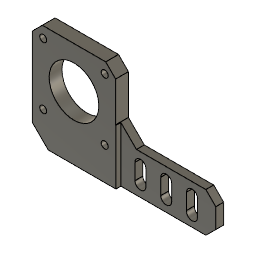
Main Assembly (Autodesk Fusion 360 archive; units mm, degrees)
design "Motor Mount"
Autodesk Fusion 360 part; units mm, degrees
sketch "Sketch1" plane through (0, 0, 0) normal (0, 1, 0) x (1, 0, 0)
  line L0 (0, 0) -> (42, 0) construction
  line L1 (42, 0) -> (42, -42) construction
  line L2 (42, -42) -> (0, -42)
  line L3 (0, -42) -> (0, 0)
  line L4 (5.5, -5.5) -> (36.5, -5.5) construction
  line L5 (36.5, -5.5) -> (36.5, -36.5) construction
  line L6 (36.5, -36.5) -> (5.5, -36.5) construction
  line L7 (5.5, -36.5) -> (5.5, -5.5) construction
  circle A0 centre (36.5, -36.5) radius 1.75
  circle A1 centre (5.5, -36.5) radius 1.75
  circle A2 centre (5.5, -5.5) radius 1.75
  circle A3 centre (36.5, -5.5) radius 1.75
  line L8 (0, -21) -> (42, -21) construction
  circle A4 centre (21, -21) radius 12.5
  line L9 (0, 0) -> (0, 11)
  line L10 (0, 11) -> (90, 11)
  line L11 (90, 11) -> (90, -9)
  line L12 (90, -9) -> (42, -9)
  line L13 (42, -9) -> (42, -42)
  line L14 (90, 1) -> (42, 1) construction
  line L15 (67.75, -3) -> (62.25, -3) construction
  line L16 (62.25, -3) -> (62.25, 5)
  line L17 (62.25, 5) -> (67.75, 5) construction
  line L18 (67.75, 5) -> (67.75, -3)
  line L19 (67.75, -3) -> (62.25, 5) construction
  line L20 (62.25, -3) -> (67.75, 5) construction
  line L21 (65, 1) -> (52, 1)
  line L22 (65, 1) -> (78, 1)
  line L23 (54.75, -3) -> (49.25, -3) construction
  line L24 (49.25, -3) -> (49.25, 5)
  line L25 (49.25, 5) -> (54.75, 5) construction
  line L26 (54.75, 5) -> (54.75, -3)
  line L27 (54.75, -3) -> (49.25, 5) construction
  line L28 (49.25, -3) -> (54.75, 5) construction
  line L29 (75.25, -3) -> (80.75, -3) construction
  line L30 (80.75, -3) -> (80.75, 5)
  line L31 (80.75, 5) -> (75.25, 5) construction
  line L32 (75.25, 5) -> (75.25, -3)
  line L33 (75.25, -3) -> (80.75, 5) construction
  line L34 (80.75, -3) -> (75.25, 5) construction
  arc A5 (54.75, 5) -> (49.25, 5) centre (52, 5) ccw
  arc A6 (49.25, -3) -> (54.75, -3) centre (52, -3) ccw
  arc A7 (67.75, 5) -> (62.25, 5) centre (65, 5) ccw
  arc A8 (62.25, -3) -> (67.75, -3) centre (65, -3) ccw
  arc A9 (75.25, -3) -> (80.75, -3) centre (78, -3) ccw
  arc A10 (80.75, 5) -> (75.25, 5) centre (78, 5.3653) ccw
  point P0 (65, 1)
  point P1 (52, 1)
  point P2 (78, 1)
  dimension "d1" = 42
  dimension "d2" = 42
  dimension "d3" = 5.5
  dimension "d4" = 3.5
  dimension "d5" = 3.5
  dimension "d6" = 3.5
  dimension "d7" = 3.5
  dimension "d12" = 11
  dimension "d13" = 90
  dimension "d14" = 20
  dimension "d15" = 5.5
  dimension "d16" = 13
  dimension "d17" = 13
  dimension "d18" = 5.5
  dimension "d19" = 8
  dimension "d20" = 5.5
  dimension "d21" = 8
  dimension "d24" = 25
  constraint horizontal L0
  constraint vertical L1
  constraint horizontal L2
  constraint vertical L3
  constraint coincident L0.start L3.end
  constraint coincident L5.end L6.start
  constraint coincident L6.end L7.start
  constraint coincident L4.start L7.end
  constraint coincident L4.end L5.start
  constraint midpoint L3 L8.start
  constraint midpoint L1 L8.end
  constraint midpoint L8 A4.centre
  constraint perpendicular L0 L9
  constraint perpendicular L9 L10
  constraint perpendicular L10 L11
  constraint coincident L1 L12.end
  constraint perpendicular L1 L12
  constraint midpoint L11 L14.start
  constraint perpendicular L11 L14
  constraint horizontal L15
  constraint perpendicular L15 L16
  constraint parallel L15 L17
  constraint parallel L16 L18
  constraint coincident L19 P0
  constraint coincident L20 P0
  constraint coincident L14 P0
  constraint coincident P0 L21.start
  constraint perpendicular L16 L21
  constraint perpendicular L18 L22
  constraint horizontal L23
  constraint perpendicular L23 L24
  constraint parallel L23 L25
  constraint parallel L24 L26
  constraint coincident L27 P1
  constraint coincident L28 P1
  constraint coincident P1 L21.end
  constraint horizontal L29
  constraint perpendicular L29 L30
  constraint parallel L29 L31
  constraint parallel L30 L32
  constraint coincident L33 P2
  constraint coincident L34 P2
  constraint coincident P2 L22.end
  constraint tangent L26 A5
  constraint tangent L26 A6
  constraint tangent L18 A7
  constraint tangent L18 A8
  constraint tangent L30 A9
  measures "d1" distance of L0.start L0.end
  measures "d2" distance of L0.start L2.end
  measures "d4" diameter of A0
  measures "d5" diameter of A1
  measures "d6" diameter of A2
  measures "d7" diameter of A3
  measures "d12" distance of L0.start L9.end
  measures "d13" distance of L9.end L10.end
  measures "d14" distance of L10.end L11.end
  measures "d15" distance of L16.end L17.end
  measures "d16" distance of P0 P1
  measures "d17" distance of P0 P2
  measures "d18" distance of L24.end L25.end
  measures "d19" distance of L23.end L24.end
  measures "d20" distance of L30.end L31.end
  measures "d21" distance of L29.end L30.end
  measures "d24" diameter of A4
extrude "Extrude1" add sketch "Sketch1" along normal blind 6.5
chamfer "Chamfer1" distance 8 angle 45 2 edges at (42, 3.25, 9) (0, 3.25, -11)
chamfer "Chamfer2" distance 5 angle 45 4 edges at (90, 3.25, 9) (90, 3.25, -11) (42, 3.25, 42) (0, 3.25, 42)
sketch "Sketch2" plane through (0, 0, -11) normal (0, 0, -1) x (1, 0, 0)
  line L0 (85, -6.5) -> (85, 0)
  line L1 (85, 0) -> (8, 0)
  line L2 (8, 0) -> (8, -6.5)
  line L3 (8, -6.5) -> (85, -6.5)
  line L4 (90, 0) -> (42.1425, 0)
  line L5 (42.1425, 0) -> (42.1425, -2.5)
  line L6 (42.1425, -2.5) -> (90, -2.5)
  line L7 (90, -2.5) -> (90, 0)
  dimension "d25" = 2.5
  constraint horizontal L4
  constraint vertical L5
  constraint horizontal L6
  constraint vertical L7
  measures "d25" distance of L4.start L6.end
extrude "Extrude3" cut sketch "Sketch2" against normal blind 36 contours L0 L1 L4 L5 L6 | L0 L4 L6 L7
equation "d25 = 6.5 mm - 4 mm"

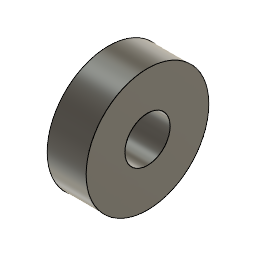
design "Bearing"
Autodesk Fusion 360 part; units mm, degrees
sketch "Sketch1" plane through (0, 0, 0) normal (1, 0, 0) x (0, 1, 0)
  circle A0 centre (0, 0) radius 11
  dimension "d1" = 22
  constraint coincident A0.centre origin
  measures "d1" diameter of A0
extrude "Extrude1" add sketch "Sketch1" along normal blind 7
sketch "Sketch2" plane through (7, 0, 0) normal (1, 0, 0) x (0, 1, 0)
  circle A0 centre (0, 0) radius 11
  circle A1 centre (0, 0) radius 4.05
  dimension "d4" = 8.1
  constraint concentric A0 A1
  measures "d4" diameter of A1
extrude "Extrude2" cut sketch "Sketch2" against normal blind 30 contours A1

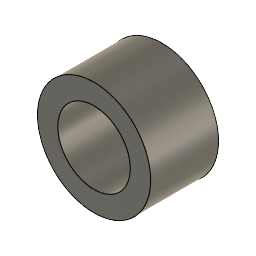
design "Bushings"
Autodesk Fusion 360 part; units mm, degrees
sketch "Sketch1" plane through (0, 0, 0) normal (0, 1, 0) x (1, 0, 0)
  circle A0 centre (0, 0) radius 4
  circle A1 centre (0, 0) radius 6.25
  dimension "d1" = 8
  dimension "d2" = 12.5
  constraint coincident A0.centre A1.centre
  measures "d1" diameter of A0
  measures "d2" diameter of A1
extrude "Extrude1" add sketch "Sketch1" along normal blind 7.5
equation "d3 = 5.75 mm + 1.75 mm"

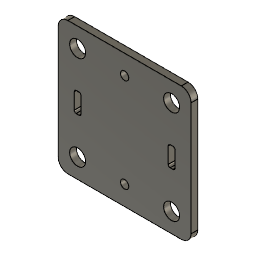
design "Gantry Plate"
Autodesk Fusion 360 part; units mm, degrees
sketch "Sketch1" plane through (0, 0, 0) normal (0, 1, 0) x (1, 0, 0)
  line L0 (0, 0) -> (48.25, 0) construction
  line L1 (48.25, 0) -> (48.25, -48.25) construction
  line L2 (48.25, -48.25) -> (0, -48.25) construction
  line L3 (0, -48.25) -> (0, 0) construction
  line L4 (-5, 10) -> (53.25, 10)
  line L5 (58.25, 5) -> (58.25, -53.25)
  line L6 (53.25, -58.25) -> (-5, -58.25)
  line L7 (-10, -53.25) -> (-10, 5)
  circle A0 centre (48.25, -48.25) radius 4.1
  circle A1 centre (48.25, 0) radius 4.1
  circle A2 centre (0, 0) radius 4.1
  circle A3 centre (0, -48.25) radius 4.1
  line L8 (49, -19) -> (47.5, -19)
  line L9 (46.5, -20) -> (46.5, -28.25)
  line L10 (47.5, -29.25) -> (49, -29.25)
  line L11 (50, -28.25) -> (50, -20)
  line L12 (50, -19) -> (46.5, -29.25) construction
  line L13 (46.5, -19) -> (50, -29.25) construction
  line L14 (0.75, -19) -> (-0.75, -19)
  line L15 (-1.75, -20) -> (-1.75, -28.25)
  line L16 (-0.75, -29.25) -> (0.75, -29.25)
  line L17 (1.75, -28.25) -> (1.75, -20)
  line L18 (1.75, -19) -> (-1.75, -29.25) construction
  line L19 (-1.75, -19) -> (1.75, -29.25) construction
  arc A4 (-10, -53.25) -> (-5, -58.25) centre (-5, -53.25) ccw
  arc A5 (53.25, -58.25) -> (58.25, -53.25) centre (53.25, -53.25) ccw
  arc A6 (58.25, 5) -> (53.25, 10) centre (53.25, 5) ccw
  arc A7 (-5, 10) -> (-10, 5) centre (-5, 5) ccw
  arc A8 (-1.75, -28.25) -> (-0.75, -29.25) centre (-0.75, -28.25) ccw
  arc A9 (0.75, -29.25) -> (1.75, -28.25) centre (0.75, -28.25) ccw
  arc A10 (1.75, -20) -> (0.75, -19) centre (0.75, -20) ccw
  arc A11 (-0.75, -19) -> (-1.75, -20) centre (-0.75, -20) ccw
  arc A12 (46.5, -28.25) -> (47.5, -29.25) centre (47.5, -28.25) ccw
  arc A13 (49, -29.25) -> (50, -28.25) centre (49, -28.25) ccw
  arc A14 (50, -20) -> (49, -19) centre (49, -20) ccw
  arc A15 (47.5, -19) -> (46.5, -20) centre (47.5, -20) ccw
  point P0 (48.25, -24.125)
  point P1 (0, -24.125)
  dimension "d1" = 48.25
  dimension "d2" = 48.25
  dimension "d4" = 8.2
  dimension "d5" = 8.2
  dimension "d6" = 8.2
  dimension "d7" = 8.2
  dimension "d8" = 3.5
  dimension "d9" = 10.25
  dimension "d10" = 3.5
  dimension "d11" = 10.25
  dimension "d12" = 5
  dimension "d13" = 1
  dimension "d14" = 1
  constraint horizontal L0
  constraint vertical L1
  constraint horizontal L2
  constraint vertical L3
  constraint coincident L0.start L3.end
  constraint coincident L1.end L2.start
  constraint coincident L0.end L1.start
  constraint coincident L2.end L3.start
  constraint horizontal L8
  constraint perpendicular L8 L9
  constraint parallel L8 L10
  constraint parallel L9 L11
  constraint coincident L12 P0
  constraint coincident L13 P0
  constraint midpoint L1 P0
  constraint horizontal L14
  constraint perpendicular L14 L15
  constraint parallel L14 L16
  constraint parallel L15 L17
  constraint coincident L18 P1
  constraint coincident L19 P1
  constraint midpoint L3 P1
  constraint tangent L6 A4
  constraint tangent L7 A4
  constraint tangent L6 A5
  constraint tangent L5 A5
  constraint equal A4 A5
  constraint tangent L5 A6
  constraint tangent L4 A6
  constraint equal A4 A6
  constraint tangent L4 A7
  constraint tangent L7 A7
  constraint equal A4 A7
  constraint coincident L18.end L16
  constraint coincident L18.end L15
  constraint tangent L16 A8
  constraint tangent L15 A8
  constraint coincident L19.end L17
  constraint coincident L19.end L16
  constraint tangent L17 A9
  constraint tangent L16 A9
  constraint equal A8 A9
  constraint coincident L18.start L17
  constraint coincident L18.start L14
  constraint tangent L17 A10
  constraint tangent L14 A10
  constraint equal A8 A10
  constraint coincident L19.start L14
  constraint coincident L19.start L15
  constraint tangent L14 A11
  constraint tangent L15 A11
  constraint equal A8 A11
  constraint coincident L12.end L10
  constraint coincident L12.end L9
  constraint tangent L10 A12
  constraint tangent L9 A12
  constraint coincident L13.end L11
  constraint coincident L13.end L10
  constraint tangent L11 A13
  constraint tangent L10 A13
  constraint equal A12 A13
  constraint coincident L12.start L11
  constraint coincident L12.start L8
  constraint tangent L11 A14
  constraint tangent L8 A14
  constraint equal A12 A14
  constraint coincident L13.start L8
  constraint coincident L13.start L9
  constraint tangent L8 A15
  constraint tangent L9 A15
  constraint equal A12 A15
  measures "d1" distance of L0.start L0.end
  measures "d2" distance of L0.start L2.end
  measures "d4" diameter of A0
  measures "d5" diameter of A1
  measures "d6" diameter of A2
  measures "d7" diameter of A3
  measures "d8" distance of L12.end L13.end
  measures "d9" distance of L13.start L12.end
  measures "d10" distance of L18.end L19.end
  measures "d11" distance of L19.start L18.end
  measures "d12" radius of A4
  measures "d13" radius of A8
  measures "d14" radius of A12
extrude "Extrude1" add sketch "Sketch1" along normal blind 3.5
sketch "Sketch2" plane through (0, 0, 0) normal (0, -1, 0) x (1, 0, 0)
  circle A0 centre (0, 0) radius 4.1
  arc A1 (46.5, 20) -> (47.5, 19) centre (47.5, 20) ccw
  line L0 (46.5, 20) -> (46.5, 28.25)
  arc A2 (47.5, 29.25) -> (46.5, 28.25) centre (47.5, 28.25) ccw
  line L1 (47.5, 29.25) -> (49, 29.25)
  arc A3 (50, 28.25) -> (49, 29.25) centre (49, 28.25) ccw
  line L2 (50, 28.25) -> (50, 20)
  arc A4 (49, 19) -> (50, 20) centre (49, 20) ccw
  line L3 (49, 19) -> (47.5, 19)
  circle A5 centre (0, 48.25) radius 4.1
  circle A6 centre (48.25, 0) radius 4.1
  arc A7 (-1.75, 20) -> (-0.75, 19) centre (-0.75, 20) ccw
  line L4 (-1.75, 20) -> (-1.75, 28.25)
  arc A8 (-0.75, 29.25) -> (-1.75, 28.25) centre (-0.75, 28.25) ccw
  line L5 (-0.75, 29.25) -> (0.75, 29.25)
  arc A9 (1.75, 28.25) -> (0.75, 29.25) centre (0.75, 28.25) ccw
  line L6 (1.75, 28.25) -> (1.75, 20)
  arc A10 (0.75, 19) -> (1.75, 20) centre (0.75, 20) ccw
  line L7 (0.75, 19) -> (-0.75, 19)
  circle A11 centre (48.25, 48.25) radius 4.1
  arc A12 (53.25, -10) -> (58.25, -5) centre (53.25, -5) ccw
  line L8 (58.25, -5) -> (58.25, 53.25)
  arc A13 (58.25, 53.25) -> (53.25, 58.25) centre (53.25, 53.25) ccw
  line L9 (53.25, 58.25) -> (-5, 58.25)
  arc A14 (-5, 58.25) -> (-10, 53.25) centre (-5, 53.25) ccw
  line L10 (-10, 53.25) -> (-10, -5)
  arc A15 (-10, -5) -> (-5, -10) centre (-5, -5) ccw
  line L11 (-5, -10) -> (53.25, -10)
  line L12 (0, 48.25) -> (48.25, 48.25) construction
  line L13 (48.25, 0) -> (0, 0) construction
  circle A16 centre (24.125, 0) radius 2.125
  circle A17 centre (24.125, 48.25) radius 2.125
  dimension "d17" = 4.25
  dimension "d18" = 4.25
  constraint coincident A5.centre L12.start
  constraint coincident A11.centre L12.end
  constraint coincident A6.centre L13.start
  constraint coincident A0.centre L13.end
  constraint midpoint L13 A16.centre
  constraint midpoint L12 A17.centre
  measures "d17" diameter of A16
  measures "d18" diameter of A17
extrude "Extrude2" cut sketch "Sketch2" against normal blind 21 contours A16 | A17
sketch "Sketch3" plane through (0, 0, 0) normal (0, 1, 0) x (1, 0, 0)

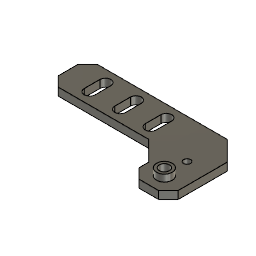
design "Idler Holder Bottom"
Autodesk Fusion 360 part; units mm, degrees
sketch "Sketch1" plane through (0, 0, 0) normal (0, 0, 1) x (1, 0, 0)
  line L0 (0, 0) -> (0, -20)
  line L1 (0, 0) -> (81, 0)
  line L2 (81, 0) -> (81, -40)
  line L3 (81, -40) -> (61, -40)
  line L4 (0, -20) -> (61, -20)
  line L5 (61, -20) -> (61, -40)
  line L6 (71, -40) -> (71, 0)
  circle A0 centre (71, -32) radius 2.6
  line L7 (0, -10) -> (61, -10) construction
  line L8 (27.75, -6) -> (33.25, -6) construction
  line L9 (33.25, -6) -> (33.25, -14)
  line L10 (33.25, -14) -> (27.75, -14) construction
  line L11 (27.75, -14) -> (27.75, -6)
  line L12 (27.75, -6) -> (33.25, -14) construction
  line L13 (33.25, -6) -> (27.75, -14) construction
  line L14 (17.75, -6) -> (12.25, -6) construction
  line L15 (12.25, -6) -> (12.25, -14)
  line L16 (12.25, -14) -> (17.75, -14) construction
  line L17 (17.75, -14) -> (17.75, -6)
  line L18 (17.75, -6) -> (12.25, -14) construction
  line L19 (12.25, -6) -> (17.75, -14) construction
  line L20 (48.75, -6) -> (43.25, -6) construction
  line L21 (43.25, -6) -> (43.25, -14)
  line L22 (43.25, -14) -> (48.75, -14) construction
  line L23 (48.75, -14) -> (48.75, -6)
  line L24 (48.75, -6) -> (43.25, -14) construction
  line L25 (43.25, -6) -> (48.75, -14) construction
  arc A1 (17.75, -6) -> (12.25, -6) centre (15, -6) ccw
  arc A2 (33.25, -6) -> (27.75, -6) centre (30.5, -6) ccw
  arc A3 (48.75, -6) -> (43.25, -6) centre (46, -6) ccw
  arc A4 (43.25, -14) -> (48.75, -14) centre (46, -14) ccw
  arc A5 (27.75, -14) -> (33.25, -14) centre (30.5, -14) ccw
  arc A6 (12.25, -14) -> (17.75, -14) centre (15, -14) ccw
  point P0 (30.5, -10)
  point P1 (15, -10)
  point P2 (46, -10)
  dimension "d1" = 20
  dimension "d2" = 81
  dimension "d3" = 40
  dimension "d4" = 20
  dimension "d5" = 61
  dimension "d11" = 5.2
  dimension "d12" = 32
  dimension "d16" = 5.5
  dimension "d17" = 8
  dimension "d18" = 5.5
  dimension "d19" = 5.5
  dimension "d20" = 8
  dimension "d23" = 34.509
  dimension "d24" = 10
  dimension "d25" = 10
  constraint coincident L0.start L1.start
  constraint vertical L0
  constraint perpendicular L0 L1
  constraint perpendicular L1 L2
  constraint perpendicular L2 L3
  constraint perpendicular L0 L4
  constraint midpoint L3 L6.start
  constraint coincident L1 L6.end
  constraint perpendicular L1 L6
  constraint coincident L6 A0.centre
  constraint midpoint L0 L7.start
  constraint perpendicular L2 L7
  constraint horizontal L8
  constraint perpendicular L8 L9
  constraint parallel L8 L10
  constraint parallel L9 L11
  constraint coincident L12 P0
  constraint coincident L13 P0
  constraint midpoint L7 P0
  constraint horizontal L14
  constraint perpendicular L14 L15
  constraint parallel L14 L16
  constraint parallel L15 L17
  constraint coincident L18 P1
  constraint coincident L19 P1
  constraint coincident L7 P1
  constraint horizontal L20
  constraint perpendicular L20 L21
  constraint parallel L20 L22
  constraint parallel L21 L23
  constraint coincident L24 P2
  constraint coincident L25 P2
  constraint coincident L7 P2
  constraint vertical L4.end L7.end
  constraint tangent L17 A1
  constraint tangent L9 A2
  constraint tangent L23 A3
  constraint tangent L23 A4
  constraint tangent L9 A5
  constraint tangent L17 A6
  measures "d1" distance of L0.start L0.end
  measures "d2" distance of L0.start L1.end
  measures "d3" distance of L1.end L2.end
  measures "d4" distance of L2.end L3.end
  measures "d5" distance of L0.end L4.end
  measures "d11" diameter of A0
  measures "d12" distance of L1 A0.centre
  measures "d16" distance of L9.end L10.end
  measures "d17" distance of L8.end L9.end
  measures "d18" distance of L15.end L16.end
  measures "d19" distance of L21.end L22.end
  measures "d20" distance of L20.end L21.end
  measures "d23" angle of L0 L18
  measures "d24" distance of L11 L17
  measures "d25" distance of L9 L21
extrude "Extrude1" add sketch "Sketch1" along normal blind 4 contours L0 L1 L3 L4 L5 L6 A0 | L1 L2 L3 L6 A0
sketch "Sketch4" plane through (0, 0, 4) normal (0, 0, 1) x (-1, 0, 0)
  circle A0 centre (-71, 32) radius 2.6
  line L0 (0, 0) -> (0, 20)
  line L1 (0, 20) -> (-61, 20)
  line L2 (-61, 20) -> (-61, 40)
  line L3 (-61, 40) -> (-81, 40)
  line L4 (-81, 40) -> (-81, 0)
  line L5 (-81, 0) -> (0, 0)
  circle A1 centre (-71, 32) radius 4
  arc A2 (-43.25, 14) -> (-48.75, 14) centre (-46, 14) ccw
  line L6 (-43.25, 14) -> (-43.25, 6)
  arc A3 (-48.75, 6) -> (-43.25, 6) centre (-46, 6) ccw
  line L7 (-48.75, 6) -> (-48.75, 14)
  arc A4 (-33.25, 6) -> (-27.75, 6) centre (-30.5, 6) ccw
  line L8 (-33.25, 6) -> (-33.25, 14)
  arc A5 (-27.75, 14) -> (-33.25, 14) centre (-30.5, 14) ccw
  line L9 (-27.75, 14) -> (-27.75, 6)
  arc A6 (-12.25, 14) -> (-17.75, 14) centre (-15, 14) ccw
  line L10 (-12.25, 14) -> (-12.25, 6)
  arc A7 (-17.75, 6) -> (-12.25, 6) centre (-15, 6) ccw
  line L11 (-17.75, 6) -> (-17.75, 14)
  dimension "d13" = 8
  constraint concentric A0 A1
  measures "d13" diameter of A1
extrude "Extrude3" add sketch "Sketch4" along normal blind 3.5 contours A1
chamfer "Chamfer1" distance 10 angle 45 2 edges at (61, -20, 2) (81, 0, 2)
chamfer "Chamfer2" distance 5 angle 45 4 edges at (81, -40, 2) (61, -40, 2) (0, -20, 2) (0, 0, 2)
sketch "Sketch5" plane through (0, 0, 4) normal (0, 0, 1) x (-1, 0, 0)
  line L0 (-5, 0) -> (0, 5)
  line L1 (0, 5) -> (0, 15)
  line L2 (0, 15) -> (-5, 20)
  line L3 (-5, 20) -> (-51, 20)
  line L4 (-51, 20) -> (-61, 30)
  line L5 (-61, 30) -> (-61, 35)
  line L6 (-61, 35) -> (-66, 40)
  line L7 (-66, 40) -> (-76, 40)
  line L8 (-76, 40) -> (-81, 35)
  line L9 (-81, 35) -> (-81, 10)
  line L10 (-81, 10) -> (-71, 0)
  line L11 (-71, 0) -> (-5, 0)
  circle A0 centre (-71, 32) radius 4
  arc A1 (-43.25, 14) -> (-48.75, 14) centre (-46, 14) ccw
  line L12 (-43.25, 14) -> (-43.25, 6)
  arc A2 (-48.75, 6) -> (-43.25, 6) centre (-46, 6) ccw
  line L13 (-48.75, 6) -> (-48.75, 14)
  arc A3 (-33.25, 6) -> (-27.75, 6) centre (-30.5, 6) ccw
  line L14 (-33.25, 6) -> (-33.25, 14)
  arc A4 (-27.75, 14) -> (-33.25, 14) centre (-30.5, 14) ccw
  line L15 (-27.75, 14) -> (-27.75, 6)
  arc A5 (-12.25, 14) -> (-17.75, 14) centre (-15, 14) ccw
  line L16 (-12.25, 14) -> (-12.25, 6)
  arc A6 (-17.75, 6) -> (-12.25, 6) centre (-15, 6) ccw
  line L17 (-17.75, 6) -> (-17.75, 14)
  line L18 (-51, 20) -> (-81, 20)
  circle A7 centre (-70.5, 20) radius 1.75
  dimension "d28" = 3.5
  dimension "d29" = 10.5
  constraint coincident L3.end L4.start
  constraint coincident L9 L18.end
  constraint perpendicular L9 L18
  constraint coincident L18 A7.centre
  measures "d28" diameter of A7
  measures "d29" distance of L9 A7.centre
extrude "Extrude4" cut sketch "Sketch5" against normal blind 10 contours L18 A7 | L18 A7
equation "d14 = 2.1 mm + 1.4 mm"

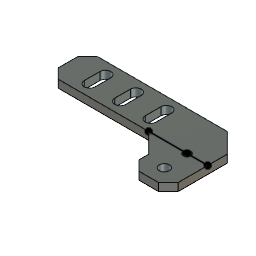
design "Idler Holder Top"
Autodesk Fusion 360 part; units mm, degrees
sketch "Sketch1" plane through (0, 0, 0) normal (0, 0, 1) x (1, 0, 0)
  line L0 (0, 0) -> (0, -20)
  line L1 (0, 0) -> (81, 0)
  line L2 (81, 0) -> (81, -40)
  line L3 (81, -40) -> (61, -40)
  line L4 (0, -20) -> (61, -20)
  line L5 (61, -20) -> (61, -40)
  line L6 (71, -40) -> (71, 0)
  circle A0 centre (71, -32) radius 2.6
  line L7 (0, -10) -> (61, -10) construction
  line L8 (27.75, -6) -> (33.25, -6) construction
  line L9 (33.25, -6) -> (33.25, -14)
  line L10 (33.25, -14) -> (27.75, -14) construction
  line L11 (27.75, -14) -> (27.75, -6)
  line L12 (27.75, -6) -> (33.25, -14) construction
  line L13 (33.25, -6) -> (27.75, -14) construction
  line L14 (17.75, -6) -> (12.25, -6) construction
  line L15 (12.25, -6) -> (12.25, -14)
  line L16 (12.25, -14) -> (17.75, -14) construction
  line L17 (17.75, -14) -> (17.75, -6)
  line L18 (17.75, -6) -> (12.25, -14) construction
  line L19 (12.25, -6) -> (17.75, -14) construction
  line L20 (48.75, -6) -> (43.25, -6) construction
  line L21 (43.25, -6) -> (43.25, -14)
  line L22 (43.25, -14) -> (48.75, -14) construction
  line L23 (48.75, -14) -> (48.75, -6)
  line L24 (48.75, -6) -> (43.25, -14) construction
  line L25 (43.25, -6) -> (48.75, -14) construction
  arc A1 (17.75, -6) -> (12.25, -6) centre (15, -6) ccw
  arc A2 (33.25, -6) -> (27.75, -6) centre (30.5, -6) ccw
  arc A3 (48.75, -6) -> (43.25, -6) centre (46, -6) ccw
  arc A4 (43.25, -14) -> (48.75, -14) centre (46, -14) ccw
  arc A5 (27.75, -14) -> (33.25, -14) centre (30.5, -14) ccw
  arc A6 (12.25, -14) -> (17.75, -14) centre (15, -14) ccw
  point P0 (30.5, -10)
  point P1 (15, -10)
  point P2 (46, -10)
  dimension "d1" = 20
  dimension "d2" = 81
  dimension "d3" = 40
  dimension "d4" = 20
  dimension "d5" = 61
  dimension "d11" = 5.2
  dimension "d12" = 32
  dimension "d16" = 5.5
  dimension "d17" = 8
  dimension "d18" = 5.5
  dimension "d19" = 5.5
  dimension "d20" = 8
  dimension "d23" = 34.509
  dimension "d24" = 10
  dimension "d25" = 10
  constraint coincident L0.start L1.start
  constraint vertical L0
  constraint perpendicular L0 L1
  constraint perpendicular L1 L2
  constraint perpendicular L2 L3
  constraint perpendicular L0 L4
  constraint midpoint L3 L6.start
  constraint coincident L1 L6.end
  constraint perpendicular L1 L6
  constraint coincident L6 A0.centre
  constraint midpoint L0 L7.start
  constraint perpendicular L2 L7
  constraint horizontal L8
  constraint perpendicular L8 L9
  constraint parallel L8 L10
  constraint parallel L9 L11
  constraint coincident L12 P0
  constraint coincident L13 P0
  constraint midpoint L7 P0
  constraint horizontal L14
  constraint perpendicular L14 L15
  constraint parallel L14 L16
  constraint parallel L15 L17
  constraint coincident L18 P1
  constraint coincident L19 P1
  constraint coincident L7 P1
  constraint horizontal L20
  constraint perpendicular L20 L21
  constraint parallel L20 L22
  constraint parallel L21 L23
  constraint coincident L24 P2
  constraint coincident L25 P2
  constraint coincident L7 P2
  constraint vertical L4.end L7.end
  constraint tangent L17 A1
  constraint tangent L9 A2
  constraint tangent L23 A3
  constraint tangent L23 A4
  constraint tangent L9 A5
  constraint tangent L17 A6
  measures "d1" distance of L0.start L0.end
  measures "d2" distance of L0.start L1.end
  measures "d3" distance of L1.end L2.end
  measures "d4" distance of L2.end L3.end
  measures "d5" distance of L0.end L4.end
  measures "d11" diameter of A0
  measures "d12" distance of L1 A0.centre
  measures "d16" distance of L9.end L10.end
  measures "d17" distance of L8.end L9.end
  measures "d18" distance of L15.end L16.end
  measures "d19" distance of L21.end L22.end
  measures "d20" distance of L20.end L21.end
  measures "d23" angle of L0 L18
  measures "d24" distance of L11 L17
  measures "d25" distance of L9 L21
extrude "Extrude1" add sketch "Sketch1" along normal blind 4 contours L0 L1 L3 L4 L5 L6 A0 | L1 L2 L3 L6 A0
sketch "Sketch4" plane through (0, 0, 4) normal (0, 0, 1) x (-1, 0, 0)
  circle A0 centre (-71, 32) radius 2.6
  line L0 (0, 0) -> (0, 20)
  line L1 (0, 20) -> (-61, 20)
  line L2 (-61, 20) -> (-61, 40)
  line L3 (-61, 40) -> (-81, 40)
  line L4 (-81, 40) -> (-81, 0)
  line L5 (-81, 0) -> (0, 0)
  circle A1 centre (-71, 32) radius 4
  arc A2 (-43.25, 14) -> (-48.75, 14) centre (-46, 14) ccw
  line L6 (-43.25, 14) -> (-43.25, 6)
  arc A3 (-48.75, 6) -> (-43.25, 6) centre (-46, 6) ccw
  line L7 (-48.75, 6) -> (-48.75, 14)
  arc A4 (-33.25, 6) -> (-27.75, 6) centre (-30.5, 6) ccw
  line L8 (-33.25, 6) -> (-33.25, 14)
  arc A5 (-27.75, 14) -> (-33.25, 14) centre (-30.5, 14) ccw
  line L9 (-27.75, 14) -> (-27.75, 6)
  arc A6 (-12.25, 14) -> (-17.75, 14) centre (-15, 14) ccw
  line L10 (-12.25, 14) -> (-12.25, 6)
  arc A7 (-17.75, 6) -> (-12.25, 6) centre (-15, 6) ccw
  line L11 (-17.75, 6) -> (-17.75, 14)
  dimension "d13" = 8
  constraint concentric A0 A1
  measures "d13" diameter of A1
chamfer "Chamfer1" distance 10 angle 45 2 edges at (61, -20, 2) (81, 0, 2)
chamfer "Chamfer2" distance 5 angle 45 4 edges at (81, -40, 2) (61, -40, 2) (0, -20, 2) (0, 0, 2)
extrude "Extrude4" add sketch "Sketch4" against normal blind 7.5 contours A1
sketch "Sketch5" plane through (0, 0, 4) normal (0, 0, 1) x (-1, 0, 0)
  circle A0 centre (-71, 32) radius 2.6
  line L0 (-5, 0) -> (0, 5)
  line L1 (0, 5) -> (0, 15)
  line L2 (0, 15) -> (-5, 20)
  line L3 (-5, 20) -> (-51, 20)
  line L4 (-51, 20) -> (-61, 30)
  line L5 (-61, 30) -> (-61, 35)
  line L6 (-61, 35) -> (-66, 40)
  line L7 (-66, 40) -> (-76, 40)
  line L8 (-76, 40) -> (-81, 35)
  line L9 (-81, 35) -> (-81, 10)
  line L10 (-81, 10) -> (-71, 0)
  line L11 (-71, 0) -> (-5, 0)
  arc A1 (-43.25, 14) -> (-48.75, 14) centre (-46, 14) ccw
  line L12 (-43.25, 14) -> (-43.25, 6)
  arc A2 (-48.75, 6) -> (-43.25, 6) centre (-46, 6) ccw
  line L13 (-48.75, 6) -> (-48.75, 14)
  arc A3 (-33.25, 6) -> (-27.75, 6) centre (-30.5, 6) ccw
  line L14 (-33.25, 6) -> (-33.25, 14)
  arc A4 (-27.75, 14) -> (-33.25, 14) centre (-30.5, 14) ccw
  line L15 (-27.75, 14) -> (-27.75, 6)
  arc A5 (-12.25, 14) -> (-17.75, 14) centre (-15, 14) ccw
  line L16 (-12.25, 14) -> (-12.25, 6)
  arc A6 (-17.75, 6) -> (-12.25, 6) centre (-15, 6) ccw
  line L17 (-17.75, 6) -> (-17.75, 14)
  line L18 (-51, 20) -> (-81, 20)
  circle A7 centre (-70.5, 20) radius 1.75
  dimension "d35" = 3.5
  dimension "d36" = 10.5
  constraint coincident L3.end L4.start
  constraint coincident L9 L18.end
  constraint perpendicular L9 L18
  constraint coincident L18 A7.centre
  measures "d35" diameter of A7
  measures "d36" distance of L9 A7.centre
extrude "Extrude6" cut sketch "Sketch5" against normal blind 11 contours L18 A7 | L18 A7
equation "d28 = -7.800 mm + 1.7 mm - 1.4 mm"

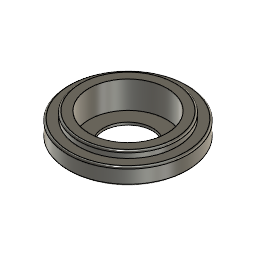
design "T-Slot Roller Wheel"
Autodesk Fusion 360 part; units mm, degrees
sketch "Sketch1" plane through (0, 0, 0) normal (0, 0, 1) x (1, 0, 0)
  circle A0 centre (0, 0) radius 11.1
  circle A1 centre (0, 0) radius 14
  dimension "d1" = 22.2
  dimension "d2" = 28
  constraint coincident A0.centre A1.centre
  measures "d1" diameter of A0
  measures "d2" diameter of A1
extrude "Extrude1" add sketch "Sketch1" along normal blind 8.5
sketch "Sketch2" plane through (0, 0, 8.5) normal (0, 0, 1) x (-1, 0, 0)
  circle A0 centre (0, 0) radius 11.1
  circle A1 centre (0, 0) radius 14
  circle A2 centre (0, 0) radius 17
  dimension "d5" = 34
  constraint concentric A0 A2
  measures "d5" diameter of A2
extrude "Extrude2" add sketch "Sketch2" against normal blind 4.75 from surface at -1.875 contours A2
sketch "Sketch3" plane through (0, 0, 0) normal (0, 0, -1) x (1, 0, 0)
  circle A0 centre (0, 0) radius 11.1
  circle A1 centre (0, 0) radius 14
  circle A2 centre (0, 0) radius 11.05
  circle A3 centre (0, 0) radius 7
  constraint coincident A0.centre A1.centre
  constraint concentric A2 A3
extrude "Extrude3" add sketch "Sketch3" against normal blind 0.75 contours A0 | A2
fillet "Fillet1" radius 0.5 4 edges at (15.8496, -6.1475, 1.875) (-13.0526, -5.0626, 0) (15.8496, 6.1475, 6.625) (-13.0526, -5.0626, 8.5)
equation "d2 = 22 mm + 6 mm"
equation "d5 = 22 mm + 6 mm + 6 mm"

design "Print Optimized IR waxer Hook"
Autodesk Fusion 360 part; units mm, degrees
sketch "Sketch1" plane through (0, 0, 0) normal (0, 1, 0) x (1, 0, 0)
  circle A0 centre (0, 0) radius 14.5 construction
  circle A1 centre (0, 0) radius 17.5 construction
  arc A2 (17.4254, -1.6143) -> (0, 17.5) centre (0, 0) ccw
  line L0 (17.4254, -1.6143) -> (-17.4254, -1.6143) construction
  arc A3 (14.4099, -1.6143) -> (-14.4099, -1.6143) centre (0, 0) ccw
  arc A4 (14.4099, -1.6143) -> (17.4254, -1.6143) centre (15.9176, -0.2341) ccw
  line L1 (-14.4099, -1.6143) -> (-14.4099, -16.6143)
  line L2 (-14.4099, -16.6143) -> (-18.4099, -16.6143)
  line L3 (-18.4099, -16.6143) -> (-18.4099, 1.5)
  line L4 (-2.4099, 17.5) -> (0, 17.5)
  arc A5 (-2.4099, 17.5) -> (-18.4099, 1.5) centre (-2.4099, 1.5) ccw
  dimension "d1" = 29
  dimension "d2" = 3
  dimension "d19" = 15
  dimension "d25" = 16
  dimension "d30" = 4
  constraint coincident A0.centre A1.centre
  constraint coincident A1 A2.end
  constraint coincident A1 A2.start
  constraint coincident A1 L0.end
  constraint horizontal L0
  constraint coincident A0 A3.end
  constraint coincident L0 A3.end
  constraint coincident A0 A3.start
  constraint coincident L0 A3.start
  constraint perpendicular L0 L1
  constraint perpendicular L1 L2
  constraint perpendicular L2 L3
  constraint tangent A1 L4
  constraint tangent L3 A5
  constraint tangent L4 A5
  measures "d1" diameter of A0
  measures "d19" distance of A3.end L1.end
  measures "d25" radius of A5
  measures "d30" distance of L1 L3
extrude "Extrude1" add sketch "Sketch1" along normal blind 100
sketch "Sketch4" plane through (-14.4099, 0, 0) normal (1, 0, 0) x (0, 1, 0)
  line L0 (0, 16.6143) -> (0, 1.6143)
  line L1 (0, 1.6143) -> (100, 1.6143)
  line L2 (100, 1.6143) -> (100, 16.6143)
  line L3 (100, 16.6143) -> (0, 16.6143)
  line L4 (0, 1.6143) -> (43.0523, 16.6143)
  line L5 (100, 1.6143) -> (61.0523, 16.6143)
  dimension "d31" = 18
  constraint coincident L0.end L1.start
  constraint coincident L3 L4.end
  constraint coincident L1.end L2.start
  constraint coincident L3 L5.end
  measures "d31" distance of L4.end L5.end
extrude "Extrude3" cut sketch "Sketch4" against normal blind 24 contours L0 L3 L4 | L2 L3 L5
sketch "Sketch5" plane through (-14.4099, 0, 0) normal (1, 0, 0) x (0, 1, 0)
  line L0 (100, 1.6143) -> (61.0523, 16.6143)
  line L1 (61.0523, 16.6143) -> (43.0523, 16.6143)
  line L2 (43.0523, 16.6143) -> (0, 1.6143)
  line L3 (0, 1.6143) -> (100, 1.6143)
  line L4 (43.0523, 16.6143) -> (43.0523, 22.6143)
  line L5 (43.0523, 22.6143) -> (33.0523, 40.6143)
  line L6 (33.0523, 40.6143) -> (71.0523, 40.6143)
  line L7 (61.0523, 16.6143) -> (61.0523, 22.6143)
  line L8 (61.0523, 22.6143) -> (71.0523, 40.6143)
  dimension "d34" = 6
  dimension "d35" = 6
  dimension "d36" = 24
  dimension "d37" = 10
  dimension "d38" = 10
  constraint coincident L1.end L2.start
  constraint perpendicular L1 L4
  constraint parallel L1 L6
  constraint coincident L0.end L1.start
  constraint perpendicular L1 L7
  measures "d34" distance of L0.end L7.end
  measures "d35" distance of L1.end L4.end
  measures "d36" distance of L1 L6
  measures "d37" horizontal distance of L6.end L7.end
  measures "d38" horizontal distance of L4.end L5.end
extrude "Extrude4" add sketch "Sketch5" against normal blind 4 contours L1 L4 L5 L6 L7 L8

design "Rotated Wax Handle"
Autodesk Fusion 360 part; units mm, degrees
sketch "Sketch1" plane through (0, 0, 0) normal (1, 0, 0) x (0, 1, 0)
  line L0 (0, 0) -> (31, 0) construction
  line L1 (15.5, 0) -> (15.5, -15.5) construction
  arc A0 (0, 0) -> (31, 0) centre (15.5, 0) ccw
  arc A1 (-3, 0) -> (34, 0) centre (15.5, 0) ccw
  arc A2 (0, 0) -> (-3, 0) centre (-1.5, 0.0833) ccw
  arc A3 (34, 0) -> (31, 0) centre (32.5, 0.1095) ccw
  dimension "d1" = 15.5
  dimension "d2" = 31
  dimension "d3" = 3
  dimension "d4" = 1.504
  dimension "d5" = 1.5023
  dimension "d6" = 17
  dimension "d7" = 17
  constraint coincident L0.start A0.start
  constraint horizontal L0
  constraint midpoint L0 L1.start
  constraint perpendicular L0 L1
  constraint coincident L1.end A0
  measures "d1" distance of L1.start L1.end
  measures "d2" distance of L0.start L0.end
  measures "d4" radius of A3
  measures "d5" radius of A2
  measures "d6" distance of L1 A2.centre
  measures "d7" distance of L1 A3.centre
extrude "Extrude1" add sketch "Sketch1" along normal blind 150 makes body 1
ref_plane "WorkPlane1" through (75, 15.5083, -8.3143) normal (1, 0, 0) x (0, 1, 0)
sketch "Sketch3" plane through (75, 0, 0) normal (1, 0, 0) x (0, 1, 0)
  line L0 (0, 0) -> (31, 0) construction
  line L1 (15.5, 0) -> (15.5, 31) construction
  line L2 (15.5, 31) -> (24.5, 31)
  line L3 (24.5, 31) -> (24.5, 37)
  line L4 (24.5, 37) -> (34.5, 55)
  line L5 (34.5, 55) -> (-3.5, 55)
  line L6 (-3.5, 55) -> (6.5, 37)
  line L7 (6.5, 37) -> (6.5, 31)
  line L8 (6.5, 31) -> (15.5, 31)
  line L9 (6.5, 31) -> (24.5, 31)
  dimension "d15" = 9
  dimension "d16" = 6
  dimension "d17" = 9
  dimension "d18" = 18
  dimension "d19" = 10
  dimension "d20" = 6
  dimension "d21" = 31
  dimension "d22" = 10
  dimension "d23" = 15.5
  constraint coincident L0.start origin
  constraint horizontal L0
  constraint midpoint L0 L1.start
  constraint perpendicular L0 L1
  constraint perpendicular L1 L2
  constraint perpendicular L2 L3
  constraint perpendicular L3 L5
  constraint perpendicular L5 L7
  constraint horizontal L8
  measures "d15" distance of L1.end L2.end
  measures "d16" distance of L2.end L3.end
  measures "d17" distance of L1.end L7.end
  measures "d18" distance of L3.end L5
  measures "d19" horizontal distance of L3.end L4.end
  measures "d20" distance of L6.end L7.end
  measures "d21" distance of L0 L7.end
  measures "d22" horizontal distance of L5.end L6.end
  measures "d23" distance of L0.start L1.start
extrude "Extrude2" add sketch "Sketch3" along normal mid plane 4 separate body makes body 2
sketch "Sketch4" plane through (75, 0, 0) normal (1, 0, 0) x (0, 1, 0)
  line L0 (0, 0) -> (-3, 0)
  line L1 (-3, 0) -> (-3, 5)
  line L2 (-3, 5) -> (0, 5)
  line L3 (0, 5) -> (0, 0)
  constraint horizontal L0
  constraint vertical L1
  constraint horizontal L2
  constraint vertical L3
  constraint coincident L0.start L3.end
extrude "Extrude3" cut sketch "Sketch4" along normal mid plane 20 bodies 1
sketch "Sketch5" plane through (75, 0, 0) normal (1, 0, 0) x (0, 1, 0)
sketch "Sketch6" plane through (75, 0, 0) normal (1, 0, 0) x (0, 1, 0)
  line L0 (0, 0) -> (31, 0) construction
  line L1 (15.5, 0) -> (15.5, 15.5)
  circle A0 centre (15.5, 15.5) radius 15.5 construction
  line L2 (0, 0) -> (-1.5, 0)
  circle A1 centre (19.4132, 10.9435) radius 15.5 construction
  line L3 (6.5, 31) -> (24.5, 31) construction
  spline S0 degree 5 poles (15.5, 31) (15.0362, 30.866) (14.1205, 30.5512) (12.7828, 29.938) (11.0722, 28.8341) (9.0623, 26.9502) (7.1882, 24.5335) (5.4525, 21.5737) (3.8468, 18.1037) (2.3583, 14.1736) (0.9739, 9.8348) (-0.0588, 6.0704) (-0.7944, 3.0938) (-1.2676, 1.0424) (-1.5, 0) knots 0 0 0 0 0 0 0.1 0.2 0.3 0.4 0.5 0.6 0.7 0.8 0.9 1 1 1 1 1 1
  point P0 (7.3292, 24.5554)
  dimension "d28" = 15.5
  dimension "d29" = 31
  dimension "d30" = 1.5
  constraint coincident L0.start L2.start
  constraint horizontal L0
  constraint midpoint L0 L1.start
  constraint perpendicular L0 L1
  constraint coincident L1.end A0.centre
  constraint coincident L1.start A0
  constraint parallel L0 L2
  constraint horizontal L3
  constraint midpoint L3 S0.start
  measures "d28" distance of L1.start L1.end
  measures "d29" diameter of A1
  measures "d30" distance of L0.start L2.end
sketch "Sketch7" plane through (75, 0, 0) normal (1, 0, 0) x (0, 1, 0)
  line L0 (0, 0) -> (31, 0)
  line L1 (15.5, 0) -> (15.5, 28) construction
  line L2 (15.5, 28) -> (24.5, 28)
  line L3 (24.5, 28) -> (6.5, 28)
  line L4 (6.5, 28) -> (6.5, 31)
  line L5 (6.5, 31) -> (24.5, 31)
  line L6 (24.5, 31) -> (24.5, 28)
  dimension "d31" = 28
  dimension "d32" = 15.5
  dimension "d33" = 9
  dimension "d34" = 18
  constraint coincident L0.start origin
  constraint horizontal L0
  constraint midpoint L0 L1.start
  constraint perpendicular L0 L1
  constraint perpendicular L1 L2
  constraint horizontal L3
  constraint vertical L4
  constraint horizontal L5
  constraint vertical L6
  measures "d31" distance of L1.start L1.end
  measures "d32" distance of L1 L0.start
  measures "d33" distance of L1.end L2.end
  measures "d34" distance of L2.end L3.end
extrude "Extrude4" add sketch "Sketch7" along normal mid plane 20 bodies 2
loft "Loft1" add section 1 face at (78.3333, -1, 0) section 2 face at (71.6667, 18.5, 28) on bodies 1 2 bodies 1 2
sketch "Sketch8" plane through (0, 0, 0) normal (1, 0, 0) x (0, 1, 0)
  circle A0 centre (15.5, 0) radius 15.4467
  circle A1 centre (19.3998, 10.937) radius 15.5
  arc A2 (9.0586, 22.483) -> (0.0533, 0) centre (27.2789, 2.1401) ccw
  circle A3 centre (27.1325, 16.141) radius 15.5
  arc A4 (24.9594, 31.4879) -> (9.0586, 22.483) centre (28.46, 6.7652) ccw
  dimension "d37" = 31
  dimension "d40" = 31
  constraint tangent A1 A2
  constraint coincident A1 A2.start
  constraint coincident A0 A2.end
  constraint tangent A3 A4
  constraint coincident A3 A4.start
  measures "d37" diameter of A1
  measures "d40" diameter of A3
extrude "Extrude5" cut sketch "Sketch8" along normal blind 150 contours A0 A1 | A0 A1 A2 | A0 A1 A3 | A0 A1 A3 | A0 A1 A3 | A0 A1 A3 | A0 A3 bodies 1
extrude "Extrude6" cut sketch "Sketch8" along normal blind 150 contours A0 A1 | A0 A1 A2 | A0 A1 A3 | A0 A1 A3 | A1 A3 A4 | A0 A1 A3 | A0 A3 | A1 A3 picked at (9.1033, 16.8285) picked at (7.4724, 10.1235) picked at (16.4185, 21.7799) bodies 1
sketch "Sketch9" plane through (85, 0, 0) normal (1, 0, 0) x (0, 1, 0)
  arc A0 (22.4484, 31) -> (9.0586, 22.483) centre (28.46, 6.7652) ccw
  line L0 (22.4484, 31) -> (6.5, 31)
  line L1 (6.5, 31) -> (6.5, 28)
  line L2 (6.5, 28) -> (-2.6396, 1.0622)
  arc A1 (0, 0) -> (-2.6396, 1.0622) centre (-1.5, 0.0833) ccw
  line L3 (0, 0) -> (0.049, 0.056)
  arc A2 (9.0586, 22.483) -> (0.049, 0.056) centre (27.2789, 2.1401) ccw
  arc A3 (6.5, 31) -> (-3, 0) centre (50.9136, 0.4337) ccw
  line L4 (6.5, 31) -> (6.5, 28)
  line L5 (6.5, 28) -> (-3, 0)
  constraint coincident L0.end L1.start
  constraint coincident L1.end L2.start
extrude "Extrude7" add sketch "Sketch9" against normal blind 20 contours L1 L2 A3 L4 L5 bodies 1
equation "d1 = ( 31 / 2 ) * 1 mm"
equation "d23 = ( 31 / 2 ) * 1 mm"
